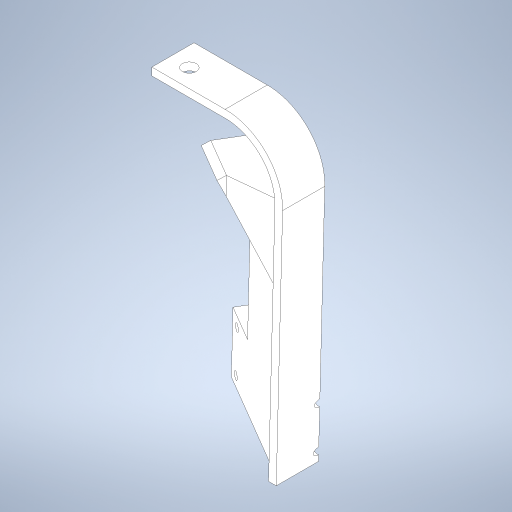
# Autodesk Inventor part: 3DOCameraMount
Saved by Autodesk Inventor 2023 (Build 270158000, 158)
## iProperties
Created: 2024-03-21
Part Number: 3DOCameraMount
Material: Generic
Document SubType Name: Modeling
Designer: incep
Density: 1 g/cm^3
Appearance: Default
Author: incep
## iProperties of the stored document 3DOCameraMount_3DPrint.ipt
Created: 2024-03-22
Part Number: 3DOCameraMount_3DPrint
Material: Generic
Document SubType Name: Modeling
Designer: incep
Density: 1 g/cm^3
Appearance: Default
Author: incep
Autodesk Inventor part; units mm, degrees
ref_plane "YZ Plane" through (0, 0, 0) normal (1, 0, 0) x (0, 1, 0)
ref_plane "XZ Plane" through (0, 0, 0) normal (0, 1, 0) x (-1, 0, 0)
sketch "Sketch1" plane through (0, 0, 0) normal (0, 0, 1) x (1, 0, 0)
  line L0 (-19, 46.892654) -> (19, 46.892654)
  line L1 (33.99486, 31.5) -> (32.345147, -31.5)
  arc A0 (33.99486, 31.5) -> (19, 46.892654) centre (19, 31.892654) ccw
  line L2 (-19, 44.892654) -> (19, 44.892654)
  arc A1 (31.995545, 31.552354) -> (19, 44.892654) centre (19, 31.892654) ccw
  line L3 (31.995545, 31.552354) -> (30.344461, -31.5)
  line L4 (-19, 46.892654) -> (-19, 44.892654)
  line L5 (30.344461, -31.5) -> (32.345147, -31.5)
  point P0 (0, 0)
  point P1 (33.170003, 0)
  point P2 (0, 46.892654)
  dimension "d0" = 88.5
  dimension "d1" = 15
  dimension "d2" = 38
  dimension "d3" = 63
  dimension "d4" = 2
  constraints: 12 end point, 4 point on circle, 2 centre point, 2 midpoint, 2 tangent, 1 horizontal, 1 horizontal alignment, 1 perpendicular, 1 vertical, 1 vertical alignment, 2 other
  measures "d0" angle of L1 L0
  measures "d1" radius of A0
  measures "d2" distance of L0.start L0.end
  measures "d3" vertical distance of L1.start L1.end
  measures "d4" radial gap between concentric circles of A0 A1
extrude "Extrusion1" add sketch "Sketch1" against normal blind 11
sketch "Sketch3" plane through (-19, 44.892654, 0) normal (0, -1, 0) x (1, 0, 0)
  line L0 (0, 0) -> (13, 0)
  line L1 (13, 0) -> (13, -14.7)
  line L2 (13, -14.7) -> (0, -14.7)
  line L3 (0, -14.7) -> (0, 0)
  line L4 (0, 0) -> (38, 0) projected
  line L5 (0, 0) -> (0, -11) projected
  point P0 (19, 0)
  dimension "d7" = 13
  dimension "d8" = 14.7
  constraints: 8 end point, 2 collinear, 2 parallel, 1 horizontal, 1 perpendicular
  measures "d7" distance of L1.end L2.end
  measures "d8" distance of L0.end L1.end
extrude "Extrusion2" [suppressed]
extrude "Extrusion3" [suppressed]
sketch "Sketch5" plane through (-19, 42.692654, 0) normal (0, -1, 0) x (1, 0, 0)
  line L0 (0, 0) -> (6.5, 0) construction
  line L1 (6.5, 0) -> (6.5, -4.77) construction
  line L2 (6.5, -4.77) -> (0, -4.77) construction
  line L3 (0, -4.77) -> (0, 0) construction
  line L4 (13, 0) -> (0, 0) construction
  line L5 (0, 0) -> (0, -14.7) construction
  circle A0 centre (6.5, -4.77) radius 1.8
  circle A1 centre (6.5, -4.77) radius 3.5
  point P0 (19, 0)
  dimension "d15" = 4.77
  dimension "d16" = 6.5
  dimension "d17" = 3.6
  dimension "d18" = 7
  constraints: 8 end point, 2 centre point, 2 coincident, 2 collinear, 2 parallel, 1 horizontal, 1 perpendicular
  measures "d15" distance of L0.end L1.end
  measures "d16" distance of L1.end L2.end
  measures "d17" diameter of A0
  measures "d18" diameter of A1
extrude "Extrusion7" [suppressed]
extrude "Extrusion8" [suppressed]
sketch "Sketch7" plane through (-19, 42.692654, 0) normal (-1, 0, 0) x (0, 0, 1)
  line L0 (-6.57, 3) -> (-2.97, 3) projected
  line L1 (-6.57, 5.2) -> (-2.97, 5.2) projected
  line L2 (-6.57, 5.2) -> (-12.7, 5.2)
  line L3 (-12.7, 5.2) -> (-12.7, 1.7)
  line L4 (-12.7, 1.7) -> (-6.57, 1.7)
  line L5 (-6.57, 1.7) -> (-6.57, 5.2)
  line L6 (0, 5.2) -> (-14.7, 5.2) projected
  line L7 (-14.7, 5.2) -> (-14.7, 0) projected
  point P0 (0, -42.692654)
  point P1 (-12.7, 3.45)
  dimension "d31" = 3.5
  dimension "d32" = 2
  constraints: 8 end point, 2 parallel, 1 collinear, 1 horizontal, 1 midpoint, 1 perpendicular, 1 point on line
  measures "d31" distance of L4.end L2.start
  measures "d32" distance from line of point (-12.7, 3.45) L7
extrude "Extrusion9" [suppressed]
sketch "Sketch8" plane through (-19, 46.892654, 0) normal (0, 1, 0) x (1, 0, 0)
  line L0 (38, 11) -> (0, 11) projected
  line L1 (13, 11) -> (18, 11)
  line L2 (18, 11) -> (18, 6.57)
  line L3 (18, 6.57) -> (13, 6.57)
  line L4 (13, 6.57) -> (13, 11)
  line L5 (13, 6.57) -> (6.5, 6.57) projected
  point P0 (19, 0)
  dimension "d35" = 5
  constraints: 8 end point, 2 parallel, 1 collinear, 1 horizontal, 1 perpendicular
  measures "d35" distance of L2.end L3.end
extrude "Extrusion10" [suppressed]
chamfer "Chamfer1" [suppressed]
sketch "Sketch9" plane through (31.995545, 31.552354, -11) normal (-0.9996573, 0.0261769, 0) x (0, 0, 1)
  line L0 (9, 0) -> (9, -63.073968)
  line L1 (11, -63.073968) -> (0, -63.073968)
  line L2 (11, 0) -> (0, 0)
  line L3 (11, 0) -> (11, -63.073968)
  point P0 (11, -32.379087)
  dimension "d41" = 2
  constraints: 2 end point, 2 point on line, 1 vertical
  measures "d41" distance between parallel lines of L3 L0
ref_plane "Work Plane1" through (31.995545, 31.552354, -2) normal (-0.4998287, 0.0130885, 0.8660254) x (-0.0261769, -0.9996573, 0)
sketch "Sketch10" plane through (31.995545, 31.552354, -2) normal (-0.4998287, 0.0130885, 0.8660254) x (-0.0261769, -0.9996573, 0)
  line L0 (47.073968, -32) -> (63.073968, -32)
  line L1 (63.073968, -32) -> (63.073968, 0)
  line L2 (63.073968, 0) -> (47.073968, 0)
  line L3 (47.073968, 0) -> (47.073968, -32)
  line L4 (63.073968, 1) -> (63.073968, -4.5)
  line L5 (0, 1) -> (63.073968, 1)
  line L6 (0, 1) -> (0, -4.5)
  line L7 (63.073968, -4.5) -> (0, -4.5)
  line L8 (63.073968, 1) -> (63.073968, -4.5)
  line L9 (0, 0) -> (63.073968, 0)
  line L10 (0.073968, -21.6) -> (47.073968, -21.6)
  line L11 (47.073968, -21.6) -> (47.073968, -10.4)
  line L12 (47.073968, -10.4) -> (0.073968, -10.4)
  line L13 (0.073968, -10.4) -> (0.073968, -21.6)
  point P0 (32.379087, -25.984171)
  point P1 (47.073968, -16)
  point P2 (47.073968, -16)
  point P3 (47.073968, -4.5)
  dimension "d43" = 32
  dimension "d44" = 16
  dimension "d45" = 11.2
  dimension "d46" = 47
  constraints: 16 end point, 4 parallel, 3 collinear, 2 horizontal, 2 midpoint, 2 perpendicular, 1 coincident
  measures "d43" distance of L0.end L1.end
  measures "d44" distance of L0.start L0.end
  measures "d45" distance between parallel lines of L10 L12
  measures "d46" distance of L10.start L10.end
extrude "Extrusion11" add sketch "Sketch10" against normal blind 4 contours L3 L7 L1 L0 | L10 L13 L12 L3 | L7 L3 L2 L1
sketch "Sketch12" plane through (23.759029, -15.32207, -10.664102) normal (0.8657286, -0.0226699, 0.5) x (0.4998287, -0.0130885, -0.8660254)
  line L0 (-4, 0) -> (-4, 47)
  line L1 (-4, 0) -> (0, 0)
  line L2 (0, 47) -> (0, 0)
  line L3 (-4, 47) -> (0, 47)
  line L4 (-4, 38.228587) -> (-4, 47)
  point P0 (-21.311369, 14.69488)
  constraints: 2 end point, 1 vertical
extrude "Extrusion13" add sketch "Sketch12" along normal up to surface surface through (33.99486, 31.5, 0) normal (0.9996573, -0.0261769, 0)
sketch "Sketch15" plane through (2.641145, -30.774563, -18) normal (-0.0261769, -0.9996573, 0) x (0.8657286, -0.0226699, 0.5)
  line L0 (29.690599, -4) -> (27.5, -7.794229)
  line L1 (27.5, -7.794229) -> (20.928203, -4)
  line L2 (10.4, -4) -> (29.690599, -4)
  line L3 (21.446961, 8.402201) -> (33, 1.732051)
  line L4 (21.446961, 8.402201) -> (15.946961, -1.124078)
  line L5 (27.5, -7.794229) -> (15.946961, -1.124078)
  line L6 (33, 1.732051) -> (27.5, -7.794229)
  point P0 (6.015829, 17.311369)
  constraints: 2 end point, 1 collinear, 1 point on line
extrude "Extrusion16" add sketch "Sketch15" against normal up to surface (63 mm away) contours L0 L1 L2
sketch "Sketch14" plane through (31.995545, 31.552354, -2) normal (-0.4998287, 0.0130885, 0.8660254) x (0.8657286, -0.0226699, 0.5)
  line L0 (-29, -49.573968) -> (-3, -49.573968) construction
  line L1 (-3, -49.573968) -> (-3, -60.573968) construction
  line L2 (-3, -60.573968) -> (-29, -60.573968) construction
  line L3 (-29, -60.573968) -> (-29, -49.573968) construction
  line L4 (-21.6, -0.073968) -> (-21.6, -47.073968) construction
  line L5 (-21.6, -47.073968) -> (-32, -47.073968) construction
  line L6 (-32, -47.073968) -> (-32, -63.073968) construction
  line L7 (-32, -63.073968) -> (0, -63.073968) construction
  line L8 (0, -0.073968) -> (0, -63.073968) construction
  circle A0 centre (-29, -49.573968) radius 0.95
  circle A1 centre (-29, -60.573968) radius 0.95
  circle A2 centre (-3, -60.573968) radius 0.95
  circle A3 centre (-3, -49.573968) radius 0.95
  line L9 (0, -0.073968) -> (-21.6, -0.073968)
  point P0 (-25.984171, -32.379087)
  point P1 (-16, -63.073968)
  point P2 (-16, -60.573968)
  point P3 (-29, -55.073968)
  point P4 (-32, -55.073968)
  dimension "d58" = 26
  dimension "d59" = 11
  dimension "d60" = 1.9
  constraints: 8 end point, 4 centre point, 4 coincident, 4 midpoint, 3 equal radius, 2 parallel, 1 horizontal, 1 horizontal alignment, 1 perpendicular, 1 vertical alignment
  measures "d58" distance of L0.start L0.end
  measures "d59" distance of L2.end L0.start
  measures "d60" diameter of A0
extrude "Extrusion15" cut sketch "Sketch14" against normal blind 20
sketch "Sketch17" plane through (12.063554, -15.015813, -12.8) normal (-0.8657286, 0.0226699, -0.5) x (-0.4998287, 0.0130885, 0.8660254)
  line L0 (0, 47) -> (0, 0)
  line L1 (0, 30) -> (7.92723, 47)
  line L2 (7.92723, 47) -> (0, 47)
  point P0 (17.311369, 14.69488)
  dimension "d67" = 17
  dimension "d68" = 25
  constraints: 4 end point, 1 horizontal, 1 point on line
  measures "d67" distance from line of L1.start L2
  measures "d68" angle of L0 L1
extrude "Extrusion17" add sketch "Sketch17" against normal up to surface (11.2 mm away)
sketch "Sketch19" plane through (12.848862, 14.973907, -12.8) normal (-0.4640615, -0.4106113, 0.7848856) x (0.8657286, -0.0226699, 0.5)
  line L0 (11.2, 0) -> (11.2, 18.757425)
  line L1 (0, 18.757425) -> (11.2, 18.757425)
  line L2 (0, 0) -> (0, 18.757425)
  line L3 (11.2, 0) -> (0, 0)
  line L4 (1, 1) -> (1, 17.757425)
  line L5 (1, 17.757425) -> (10.2, 17.757425)
  line L6 (10.2, 17.757425) -> (10.2, 1)
  line L7 (10.2, 1) -> (1, 1)
  line L8 (1, 1) -> (1, 0)
  line L9 (10.2, 1) -> (10.2, 0)
  point P0 (-4.384171, -6.555048)
  dimension "d71" = 1
  dimension "d72" = 9.2
  constraints: 12 end point, 2 perpendicular, 2 point on line, 3 other
  measures "d71" distance between parallel lines of L3 L7
  measures "d72" distance of L4.end L5.end
extrude "Extrusion18" add sketch "Sketch19" along normal blind 2 contours L3 L9 L6 L5 L4 L8 L2 L1 L0
sketch "Sketch20" plane through (13.714591, 14.951237, -12.3) normal (0.1875123, -0.9115286, -0.3659982) x (0.8657286, -0.0226699, 0.5)
  line L0 (10.2, 0) -> (9.2, 0) projected
  line L1 (10.2, 0) -> (10.2, 2) projected
  line L2 (9.2, 2) -> (10.2, 2) projected
  line L3 (9.2, 0) -> (9.2, 2) projected
  line L4 (0, 0) -> (-1, 0) projected
  line L5 (0, 0) -> (0, 2) projected
  line L6 (-1, 2) -> (0, 2) projected
  line L7 (-1, 0) -> (-1, 2) projected
  point P0 (-5.384171, 22.157652)
extrude "Extrusion19" add sketch "Sketch20" along normal up to surface surface through (14.907242, 0.281044, -11.389944) normal (-0.4998287, 0.0130885, 0.8660254)
sketch "Sketch21" plane through (-19, 46.892654, 0) normal (0, 1, 0) x (1, 0, 0)
  line L0 (52.99486, 0) -> (52.99486, 11)
  circle A0 centre (23.89486, 4.77) radius 1.8
  line L1 (38, 0) -> (0, 0)
  line L2 (38, 0) -> (0, 0)
  line L3 (38, 0) -> (38, 11)
  line L4 (0, 11) -> (38, 11)
  line L5 (0, 0) -> (0, 11)
  line L6 (18.89486, 0) -> (18.89486, 11)
  point P0 (19, 0)
  dimension "d77" = 29.1
  dimension "d78" = 3.6
  dimension "d79" = 4.77
  dimension "d80" = 5
  constraints: 2 end point, 2 point on line, 1 centre point, 1 perpendicular
  measures "d77" distance from line of A0.centre L0
  measures "d78" diameter of A0
  measures "d79" distance from line of A0.centre L1
  measures "d80" distance from line of A0.centre L6
extrude "Extrusion20" cut sketch "Sketch21" against normal up to surface (2 mm away) contours A0 | L1 L5 L4 L6
sketch "Sketch24" plane through (31.993609, 31.478411, -2) normal (0.0261769, 0.9996573, 0) x (0.9996573, -0.0261769, 0)
  line L0 (-12.970279, -1.665183) -> (-9.006664, 5.2)
  line L1 (-1.775352, 1.025) -> (-3.4208, 1.975)
  line L2 (-1.775352, 1.025) -> (-3.4208, 1.975)
  line L3 (-27.712813, 16) -> (0, 0)
  line L4 (0, 0) -> (-9.006664, 5.2)
  line L5 (0, 0) -> (-12.970279, -1.665183)
  line L6 (-9.87269, 5.7) -> (-17.840123, 10.3)
  line L7 (-12.970279, -1.665183) -> (-13.876587, -3.234954)
  line L8 (-13.876587, -3.234954) -> (-9.006664, 5.2)
  line L9 (-17.840123, 10.3) -> (-18.706149, 10.8)
  line L10 (-9.006664, 5.2) -> (-9.87269, 5.7)
  line L11 (-18.706149, 10.8) -> (-27.712813, 16)
  point P0 (-31.158637, -2)
  point P1 (-21.487547, 18.030192)
  point P2 (-22.943031, 19.251489)
  point P3 (-21.487547, 18.030192)
  point P4 (-22.943031, 19.251489)
  point P5 (0, 0)
  point P6 (-1.775352, 1.025)
  point P7 (-3.4208, 1.975)
  point P8 (-9.006664, 5.2)
  constraints: 2 end point
extrude "Extrusion22" add sketch "Sketch24" against normal up to surface surface through (15.010195, 22.574698, -4.997638) normal (-0.4640615, -0.4106113, 0.7848856)
equation "\"d68\" = zangle"
equation "\"yangle\" = 30deg"
equation "\"zangle\" = 25deg"
equation "\"d42\" = yangle"
body "Solid1"
